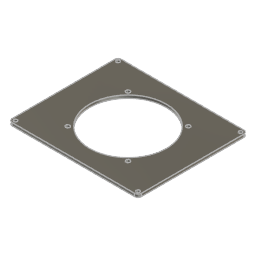
Metronome_Lid (Autodesk Fusion 360 design; units mm, degrees)
part number: 2026-07-24-11-18-37-299
Autodesk Fusion 360 part; units mm, degrees
note: some values were not read from the file. Set by a fixed rule: which sketch regions a step uses.
sketch "Sketch1" plane through (0, 0, 0) normal (0, 0, 1) x (1, 0, 0)
  line L0 (65, 55) -> (-65, 55)
  line L1 (-65, 55) -> (-65, -55)
  line L2 (-65, -55) -> (65, -55)
  line L3 (65, -55) -> (65, 55)
  line L4 (65, 55) -> (-65, -55) construction
  line L5 (-65, 55) -> (65, -55) construction
  line L6 (61.5, 51.5) -> (-61.5, 51.5)
  line L7 (-61.5, 51.5) -> (-61.5, -51.5)
  line L8 (-61.5, -51.5) -> (61.5, -51.5)
  line L9 (61.5, -51.5) -> (61.5, 51.5)
  line L10 (61.5, 51.5) -> (-61.5, -51.5) construction
  line L11 (-61.5, 51.5) -> (61.5, -51.5) construction
  circle A0 centre (-61.5, 51.5) radius 3.5
  circle A1 centre (61.5, 51.5) radius 3.5
  circle A2 centre (61.5, -51.5) radius 3.5
  circle A3 centre (-61.5, -51.5) radius 3.5
  circle A4 centre (-61.5, -51.5) radius 1.75
  circle A5 centre (61.5, -51.5) radius 1.75
  circle A6 centre (61.5, 51.5) radius 1.75
  circle A7 centre (-61.5, 51.5) radius 1.75
  circle A8 centre (0, 0) radius 38.5
  line L12 (30.25, 30.25) -> (-30.25, 30.25)
  line L13 (-30.25, 30.25) -> (-30.25, -30.25)
  line L14 (-30.25, -30.25) -> (30.25, -30.25)
  line L15 (30.25, -30.25) -> (30.25, 30.25)
  line L16 (30.25, 30.25) -> (-30.25, -30.25) construction
  line L17 (-30.25, 30.25) -> (30.25, -30.25) construction
  circle A9 centre (30.25, 30.25) radius 2
  circle A10 centre (-30.25, 30.25) radius 2
  circle A11 centre (-30.25, -30.25) radius 2
  circle A12 centre (30.25, -30.25) radius 2
  dimension "d1" = 130
  dimension "d2" = 110
  dimension "d3" = 3.5
  dimension "d4" = 3.5
  dimension "d5" = 3.5
  dimension "d6" = 3.5
  dimension "d7" = 3.5
  dimension "d8" = 3.5
  dimension "d9" = 77
  dimension "d10" = 60.5
  dimension "d11" = 60.5
  dimension "d12" = 4
  dimension "d13" = 4
  dimension "d14" = 4
  dimension "d15" = 4
  constraint horizontal L0
  constraint perpendicular L0 L1
  constraint parallel L0 L2
  constraint parallel L1 L3
  constraint coincident L4 A8.centre
  constraint coincident L5 A8.centre
  constraint coincident A8.centre origin
  constraint horizontal L6
  constraint perpendicular L6 L7
  constraint parallel L6 L8
  constraint parallel L7 L9
  constraint coincident L10 A8.centre
  constraint coincident L11 A8.centre
  constraint coincident L6.end L7.start
  constraint tangent L0 A0
  constraint coincident L6.start L9.end
  constraint tangent L0 A1
  constraint coincident L8.end L9.start
  constraint tangent L2 A2
  constraint coincident L7.end L8.start
  constraint tangent L1 A3
  constraint concentric A3 A4
  constraint concentric A2 A5
  constraint concentric A1 A6
  constraint concentric A0 A7
  constraint horizontal L12
  constraint perpendicular L12 L13
  constraint parallel L12 L14
  constraint parallel L13 L15
  constraint coincident L16 A8.centre
  constraint coincident L17 A8.centre
  constraint coincident L12.start L15.end
  constraint coincident L12.end L13.start
  constraint coincident L13.end L14.start
  constraint coincident L14.end L15.start
  measures "d1" distance of L1.end L2.end
  measures "d2" distance of L0.end L1.end
  measures "d3" distance of L3 L9
  measures "d4" distance of L0 L6
  measures "d5" diameter of A4
  measures "d6" diameter of A5
  measures "d7" diameter of A6
  measures "d8" diameter of A7
  measures "d9" diameter of A8
  measures "d10" distance of L13.end L14.end
  measures "d11" distance of L12.end L13.end
  measures "d12" diameter of A9
  measures "d13" diameter of A10
  measures "d14" diameter of A11
  measures "d15" diameter of A12
extrude "Extrude1" add sketch "Sketch1" along normal blind 3 contours L0 L6 A0 A1 | L6 L9 A1 A6 | L3 L9 A1 A2 | L6 L7 A0 A7 | L6 L7 L8 L9 A0 A1 A2 A3 | L6 L9 A1 A6 | L8 L9 A2 A5 | L6 L7 A0 A7 | L1 L7 A0 A3 | L8 L9 A2 A5 | L2 L8 A2 A3 | L7 L8 A3 A4 | L7 L8 A3 A4 | A8 L12 L15 A9 | A8 L14 L15 A12 | A8 L12 L13 A10 | A8 L13 L14 A11
